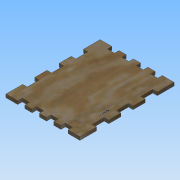
# Autodesk Inventor part: WallToWall
Saved by Autodesk Inventor 2015 (Build 190159000, 159)
## iProperties
Created: 2014-11-11
Part Number: WallToWall
Material: Generic
Document SubType Name: Modeling
Designer: 0
Density: 1 g/cm^3
Appearance: Plywood - Weathered
Mass: 154.278 g
Surface Area: 543.527 cm^2
Volume: 154.278 cm^3
Author: 0
Autodesk Inventor part; units mm, degrees
ref_plane "YZ Plane" through (0, 0, 0) normal (1, 0, 0) x (0, 1, 0)
ref_plane "XZ Plane" through (0, 0, 0) normal (0, 1, 0) x (-1, 0, 0)
ref_plane "XY Plane" through (0, 0, 0) normal (0, 0, 1) x (1, 0, 0)
sketch "Sketch1" plane through (0, 0, 0) normal (0, 1, 0) x (-1, 0, 0)
  line L0 (0, 0) -> (127, 0)
  line L1 (127, 0) -> (127, -166.624)
  line L2 (127, -166.624) -> (0, -166.624)
  line L3 (0, -166.624) -> (0, 0)
  dimension "BoxHeight" = 127
  dimension "d1" = 166.624
  constraints: 8 end point, 2 parallel, 1 coincident, 1 horizontal, 1 perpendicular
  measures "BoxHeight" distance of L1.end L2.end
  measures "d1" distance of L0.end L1.end
sketch "Sketch2" plane through (0, 0, 0) normal (0, 1, 0) x (-1, 0, 0)
  line L0 (0, 0) -> (-8.89, 0)
  line L1 (-8.89, 0) -> (-8.89, -23.8034)
  line L2 (-8.89, -23.8034) -> (0, -23.8034)
  line L3 (0, -23.8034) -> (0, 0)
  line L4 (0, -166.624) -> (0, 0) projected
  line L5 (0, 0) -> (127, 0) projected
  line L6 (0, -47.6069) -> (-8.89, -47.6069)
  line L7 (-8.89, -47.6069) -> (-8.89, -71.4103)
  line L8 (-8.89, -71.4103) -> (0, -71.4103)
  line L9 (0, -71.4103) -> (0, -47.6069)
  line L10 (0, -95.2137) -> (-8.89, -95.2137)
  line L11 (-8.89, -95.2137) -> (-8.89, -119.0171)
  line L12 (-8.89, -119.0171) -> (0, -119.0171)
  line L13 (0, -119.0171) -> (0, -95.2137)
  line L14 (63.5, 0) -> (63.5, -115.824) construction
  line L15 (127, -23.8034) -> (127, 0)
  line L16 (127, -166.624) -> (127, 0)
  line L17 (127, -71.4103) -> (127, -47.6069)
  line L18 (127, -119.0171) -> (127, -95.2137)
  line L19 (28.2222, -166.624) -> (14.1111, -166.624)
  line L20 (14.1111, -166.624) -> (14.1111, -175.514)
  line L21 (14.1111, -175.514) -> (28.2222, -175.514)
  line L22 (28.2222, -175.514) -> (28.2222, -166.624)
  line L23 (127, -166.624) -> (0, -166.624) projected
  line L24 (56.4444, -166.624) -> (42.3333, -166.624)
  line L25 (42.3333, -166.624) -> (42.3333, -175.514)
  line L26 (42.3333, -175.514) -> (56.4444, -175.514)
  line L27 (56.4444, -175.514) -> (56.4444, -166.624)
  line L28 (84.6667, -166.624) -> (70.5556, -166.624)
  line L29 (70.5556, -166.624) -> (70.5556, -175.514)
  line L30 (70.5556, -175.514) -> (84.6667, -175.514)
  line L31 (84.6667, -175.514) -> (84.6667, -166.624)
  line L32 (112.8889, -166.624) -> (98.7778, -166.624)
  line L33 (98.7778, -166.624) -> (98.7778, -175.514)
  line L34 (98.7778, -175.514) -> (112.8889, -175.514)
  line L35 (112.8889, -175.514) -> (112.8889, -166.624)
  line L36 (127, -83.312) -> (0, -83.312) construction
  line L37 (63.5, -166.624) -> (63.5, -50.8) construction
  line L38 (28.2222, 0) -> (14.1111, 0)
  line L39 (14.1111, 0) -> (14.1111, 8.89)
  line L40 (14.1111, 8.89) -> (28.2222, 8.89)
  line L41 (28.2222, 8.89) -> (28.2222, 0)
  line L42 (127, 0) -> (0, 0)
  line L43 (56.4444, 0) -> (42.3333, 0)
  line L44 (42.3333, 0) -> (42.3333, 8.89)
  line L45 (42.3333, 8.89) -> (56.4444, 8.89)
  line L46 (56.4444, 8.89) -> (56.4444, 0)
  line L47 (84.6667, 0) -> (70.5556, 0)
  line L48 (70.5556, 0) -> (70.5556, 8.89)
  line L49 (84.6667, 8.89) -> (84.6667, 0)
  line L50 (70.5556, 8.89) -> (84.6667, 8.89)
  line L51 (112.8889, 0) -> (98.7778, 0)
  line L52 (98.7778, 0) -> (98.7778, 8.89)
  line L53 (112.8889, 8.89) -> (112.8889, 0)
  line L54 (98.7778, 8.89) -> (112.8889, 8.89)
  line L55 (0, -142.8206) -> (-8.89, -142.8206)
  line L56 (-8.89, -142.8206) -> (-8.89, -159.3669)
  line L57 (-8.89, -159.3669) -> (0, -159.3669)
  line L58 (0, -159.3669) -> (0, -142.8206)
  line L59 (127, -166.624) -> (127, 0)
  line L60 (127, 0) -> (135.89, 0)
  line L61 (135.89, 0) -> (135.89, -23.8034)
  line L62 (135.89, -23.8034) -> (127, -23.8034)
  line L63 (127, -23.8034) -> (127, 0)
  line L64 (127, -166.624) -> (127, 0)
  line L65 (127, -47.6069) -> (135.89, -47.6069)
  line L66 (135.89, -47.6069) -> (135.89, -71.4103)
  line L67 (135.89, -71.4103) -> (127, -71.4103)
  line L68 (127, -71.4103) -> (127, -47.6069)
  line L69 (127, -95.2137) -> (135.89, -95.2137)
  line L70 (135.89, -95.2137) -> (135.89, -119.0171)
  line L71 (135.89, -119.0171) -> (127, -119.0171)
  line L72 (127, -119.0171) -> (127, -95.2137)
  line L73 (135.89, -142.8206) -> (135.89, -159.3669)
  line L74 (127, -142.8206) -> (135.89, -142.8206)
  line L75 (127, -159.3669) -> (127, -142.8206)
  line L76 (135.89, -159.3669) -> (127, -159.3669)
  line L77 (14.1111, -175.514) -> (0, -175.514)
  line L78 (0, -175.514) -> (0, -159.3669)
  line L79 (0, -159.3669) -> (14.1111, -159.3669)
  line L80 (14.1111, -159.3669) -> (14.1111, -175.514)
  line L81 (28.2222, -175.514) -> (42.3333, -175.514)
  line L82 (42.3333, -175.514) -> (42.3333, -166.624)
  line L83 (42.3333, -166.624) -> (28.2222, -166.624)
  line L84 (28.2222, -166.624) -> (28.2222, -175.514)
  line L85 (56.4444, -175.514) -> (70.5556, -175.514)
  line L86 (70.5556, -175.514) -> (70.5556, -166.624)
  line L87 (70.5556, -166.624) -> (56.4444, -166.624)
  line L88 (56.4444, -166.624) -> (56.4444, -175.514)
  line L89 (84.6667, -175.514) -> (98.7778, -175.514)
  line L90 (98.7778, -175.514) -> (98.7778, -166.624)
  line L91 (98.7778, -166.624) -> (84.6667, -166.624)
  line L92 (84.6667, -166.624) -> (84.6667, -175.514)
  line L93 (112.8889, -175.514) -> (127, -175.514)
  line L94 (127, -175.514) -> (127, -159.3669)
  line L95 (127, -159.3669) -> (112.8889, -159.3669)
  line L96 (112.8889, -159.3669) -> (112.8889, -175.514)
  line L97 (112.8889, 0) -> (127, 0)
  line L98 (127, 0) -> (127, 8.89)
  line L99 (127, 8.89) -> (112.8889, 8.89)
  line L100 (112.8889, 8.89) -> (112.8889, 0)
  line L101 (98.7778, 8.89) -> (84.6667, 8.89)
  line L102 (84.6667, 8.89) -> (84.6667, 0)
  line L103 (84.6667, 0) -> (98.7778, 0)
  line L104 (98.7778, 0) -> (98.7778, 8.89)
  line L105 (70.5556, 8.89) -> (56.4444, 8.89)
  line L106 (56.4444, 8.89) -> (56.4444, 0)
  line L107 (56.4444, 0) -> (70.5556, 0)
  line L108 (70.5556, 0) -> (70.5556, 8.89)
  line L109 (42.3333, 8.89) -> (28.2222, 8.89)
  line L110 (28.2222, 8.89) -> (28.2222, 0)
  line L111 (28.2222, 0) -> (42.3333, 0)
  line L112 (42.3333, 0) -> (42.3333, 8.89)
  line L113 (14.1111, 8.89) -> (0, 8.89)
  line L114 (0, 8.89) -> (0, 0)
  line L115 (0, 0) -> (14.1111, 0)
  line L116 (14.1111, 0) -> (14.1111, 8.89)
  line L117 (0, 0) -> (-8.89, 0)
  line L118 (-8.89, 0) -> (-8.89, 8.89)
  line L119 (-8.89, 8.89) -> (0, 8.89)
  line L120 (0, 8.89) -> (0, 0)
  line L121 (0, -159.3669) -> (-8.89, -159.3669)
  line L122 (-8.89, -159.3669) -> (-8.89, -168.2569)
  line L123 (-8.89, -168.2569) -> (0, -168.2569)
  line L124 (0, -168.2569) -> (0, -159.3669)
  line L125 (127, -159.3669) -> (135.89, -159.3669)
  line L126 (135.89, -159.3669) -> (135.89, -168.2569)
  line L127 (135.89, -168.2569) -> (127, -168.2569)
  line L128 (127, -168.2569) -> (127, -159.3669)
  line L129 (127, 0) -> (135.89, 0)
  line L130 (135.89, 0) -> (135.89, 8.89)
  line L131 (135.89, 8.89) -> (127, 8.89)
  line L132 (127, 8.89) -> (127, 0)
  line L133 (127, -168.2569) -> (135.89, -168.2569)
  line L134 (135.89, -168.2569) -> (135.89, -175.514)
  line L135 (135.89, -175.514) -> (127, -175.514)
  line L136 (127, -175.514) -> (127, -168.2569)
  line L137 (0, -168.2569) -> (-8.89, -168.2569)
  line L138 (-8.89, -168.2569) -> (-8.89, -175.514)
  line L139 (-8.89, -175.514) -> (0, -175.514)
  line L140 (0, -175.514) -> (0, -168.2569)
  dimension "d2" = 8.89
  dimension "d3" = 23.8034
  dimension "d5" = 8.89
  dimension "d6" = 23.8034
  dimension "d7" = 23.8034
  dimension "d8" = 8.89
  dimension "d9" = 23.8034
  dimension "d10" = 23.8034
  dimension "d11" = 14.1111
  dimension "d12" = 127
  dimension "d13" = 14.1111
  dimension "d14" = 8.89
  dimension "d15" = 8.89
  dimension "d16" = 14.1111
  dimension "d17" = 8.89
  dimension "d18" = 14.1111
  dimension "d22" = 8.89
  dimension "d23" = 14.1111
  dimension "d27" = 14.1111
  dimension "d28" = 14.1111
  dimension "d29" = 14.1111
  dimension "d34" = 8.89
  dimension "d35" = 16.5463
  dimension "d40" = 23.8034
  dimension "d41" = 8.89
  dimension "d42" = 8.89
  dimension "d43" = 8.89
  dimension "d44" = 8.89
  dimension "d45" = 8.89
  dimension "d46" = 8.89
  dimension "d47" = 8.89
  dimension "d48" = 8.89
  constraints: 276 end point, 48 parallel, 43 symmetric about line, 24 horizontal, 24 perpendicular, 9 collinear, 2 midpoint, 2 point on line, 1 vertical
  measures "d2" distance of L1.end L2.end
  measures "d3" distance of L0.end L1.end
  measures "d5" distance of L7.end L8.end
  measures "d6" distance of L6.end L7.end
  measures "d7" distance between parallel lines of L2 L6
  measures "d8" distance of L10.start L10.end
  measures "d9" distance of L10.end L11.end
  measures "d10" distance between parallel lines of L8 L10
  measures "d11" distance between parallel lines of L4 L20
  measures "d12" distance of L23.start L4.start
  measures "d13" distance of L20.end L21.end
  measures "d14" distance of L19.end L20.end
  measures "d15" distance of L24.end L25.end
  measures "d16" distance of L25.end L26.end
  measures "d17" distance of L28.end L29.end
  measures "d18" distance of L29.end L31.start
  measures "d22" distance of L32.end L33.end
  measures "d23" distance of L33.end L35.start
  measures "d27" distance between parallel lines of L25 L22
  measures "d28" distance between parallel lines of L27 L29
  measures "d29" distance between parallel lines of L31 L33
  measures "d34" distance of L55.start L56.start
  measures "d35" distance of L56.start L56.end
  measures "d40" distance between parallel lines of L12 L55
  measures "d41" distance of L118.end L119.end
  measures "d42" distance of L117.end L118.end
  measures "d43" distance of L123.end L122.end
  measures "d44" distance of L122.end L121.end
  measures "d45" distance of L126.end L127.end
  measures "d46" distance of L125.end L126.end
  measures "d47" distance of L131.end L130.end
  measures "d48" distance of L130.end L129.end
extrude "Connections" add sketch "Sketch2" along normal blind 6.35 contours L3 L2 L1 L0 | L114 L113 L39 L5 | L0 L118 L119 L114 | L4 L8 L7 L6 | L41 L109 L44 L5 | L4 L12 L11 L10 | L46 L105 L48 L5 | L4 L57 L56 L55 | L49 L101 L52 L5 | L79 L80 L23 L4 | L4 L78 L123 L122 L57 | L23 L20 L77 L78 | L53 L99 L98 L5 | L78 L139 L138 L123 | L60 L61 L62 L15 | L98 L131 L130 L60 | L23 L25 L81 L22 | L65 L66 L67 L16 | L23 L29 L85 L27 | L69 L70 L71 L16 | L23 L33 L89 L31 | L74 L73 L76 L16 | L96 L95 L16 L23 | L23 L94 L93 L35 | L76 L126 L127 L94 L16 | L94 L127 L134 L135
extrude "Base Extrusion" add sketch "Sketch1" along normal blind 6.35
sketch "Sketch3" plane through (0, 6.35, 0) normal (0, 1, 0) x (1, 0, 0)
  line L0 (-6.2788, 64.0613) -> (-6.2788, 44.7093) construction
  line L1 (-6.2788, 44.7093) -> (-46.5625, 44.7093) construction
  line L2 (-46.5625, 44.7093) -> (-46.5625, 64.0613) construction
  line L3 (-46.5625, 64.0613) -> (-6.2788, 64.0613) construction
  point P0 (0, 0)
  constraints: 2 other
sketch "Sketch4" plane through (0, 6.35, 0) normal (0, 1, 0) x (1, 0, 0)
  point P0 (0, 0)
equation "\"d1\" = BaseWidth"
equation "\"d2\" = WallConA"
equation "\"d3\" = WallConB"
equation "\"d5\" = d2"
equation "\"d6\" = WallConSpace"
equation "\"d7\" = d4"
equation "\"d8\" = d2"
equation "\"d9\" = d6"
equation "\"d10\" = d4"
equation "\"d11\" = -0.8 * d13 + 0.2 * d12"
equation "\"d13\" = 0.111111 * d12"
equation "\"d14\" = WallConA"
equation "\"d15\" = d14"
equation "\"d16\" = d13"
equation "\"d17\" = d15"
equation "\"d18\" = d20"
equation "\"d22\" = d17"
equation "\"d23\" = d25"
equation "\"d27\" = d11"
equation "\"d28\" = d27"
equation "\"d29\" = d11"
equation "\"d34\" = d36"
equation "\"d35\" = d37"
equation "\"d40\" = d7"
equation "\"d41\" = d5"
equation "\"d42\" = d5"
equation "\"d43\" = d41"
equation "\"d44\" = d42"
equation "\"d45\" = d41"
equation "\"d46\" = d42"
equation "\"d47\" = d41"
equation "\"d48\" = d42"
equation "\"d4\" = WallConSpace"
equation "\"d20\" = 0.111111 * d21"
equation "\"d25\" = 0.111111 * d26"
equation "\"d36\" = d38"
equation "\"d37\" = d39"
equation "\"BaseWidth\" = 166.624"
equation "\"WallConA\" = 8.89"
equation "\"WallConB\" = 23.803429"
equation "\"WallConSpace\" = 23.803429"
equation "\"d21\" = 127"
equation "\"d26\" = 127"
equation "\"d38\" = 8.89"
equation "\"d39\" = 16.546286"
body "Solid1"
